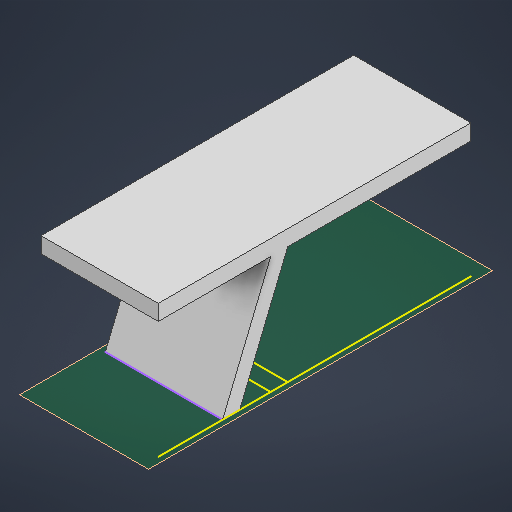
# Autodesk Inventor part: сосало
Saved by Autodesk Inventor 2025 (Build 290162000, 162)
## iProperties
Created: 2024-11-12
Part Number: сосало
Material: Типовые
Document SubType Name: Modeling
Designer: Phantom
Density: 1 g/cm^3
Appearance: По умолчанию
Author: Phantom
Autodesk Inventor part; units mm, degrees
ref_plane "YZ Plane" through (0, 0, 0) normal (1, 0, 0) x (0, 1, 0)
ref_plane "XZ Plane" through (0, 0, 0) normal (0, 1, 0) x (-1, 0, 0)
ref_plane "XY Plane" through (0, 0, 0) normal (0, 0, 1) x (1, 0, 0)
sketch "Эскиз1" plane through (0, 0, 0) normal (0, 0, 1) x (1, 0, 0)
  line L0 (0, 0) -> (-30, 0)
  line L1 (-30, 0) -> (-30, 4)
  line L2 (-30, 4) -> (0, 4)
  line L3 (0, 4) -> (0, 0)
  dimension "d0" = 30
  dimension "d1" = 4
  constraints: 8 end point, 2 parallel, 1 horizontal, 1 perpendicular
  measures "d0" distance of L1.end L2.end
  measures "d1" distance of L0.end L1.end
extrude "Выдавливание1" add sketch "Эскиз1" along normal blind 80
sketch "Эскиз2" plane through (-30, 0, 0) normal (0, -1, 0) x (1, 0, 0)
  line L0 (30, 0) -> (30, 80) projected
  line L1 (0, 0) -> (0, 80) projected
  line L2 (30, 51.2556) -> (0, 51.2556)
  line L3 (0, 51.2556) -> (0, 46.8879)
  line L4 (0, 46.8879) -> (30, 46.8879)
  line L5 (30, 46.8879) -> (30, 51.2556)
  constraints: 8 end point, 2 parallel, 2 point on line, 1 horizontal, 1 perpendicular
ref_plane "РабПлоскость1" through (-30, -30, 0) normal (0, -1, 0) x (1, 0, 0)
sketch "Эскиз3" plane through (-30, -30, 0) normal (0, -1, 0) x (1, 0, 0)
  line L0 (30, 51.2556) -> (0, 51.2556) projected
  line L1 (0, 46.8879) -> (30, 46.8879) projected
  line L2 (0, 63.5353) -> (0, 59.1677)
  line L3 (30, 63.5353) -> (30, 59.1677)
  line L4 (30, 0) -> (30, 80) projected
  line L5 (0, 59.1677) -> (30, 59.1677)
  line L6 (30, 63.5353) -> (0, 63.5353)
  constraints: 8 end point, 1 collinear, 1 parallel, 1 perpendicular, 1 vertical
sketch "Эскиз4" plane through (0, 0, 0) normal (1, 0, 0) x (0, 0, -1)
  line L0 (-51.2556, 0) -> (-63.5353, -30)
  line L1 (-46.8879, 0) -> (-59.1677, -30)
  point P0 (0, 0)
  constraints: 4 end point
sweep "Сдвиг1" add profiles "Эскиз2" path "Эскиз4" path curves L1
